Autodesk Inventor part; units mm, degrees
(part 3 of 3)
sketch "Эскиз6" plane through (0, 2, 0) normal (0, 1, 0) x (1, 0, 0)
  circle A0 centre (0, -40) radius 1.6 construction
  circle A1 centre (-46, 0) radius 1.6 construction
  circle A2 centre (46, 0) radius 1.6 construction
  line L0 (-6.2595, 46.1335) -> (-19.2746, 46.1335) construction
  arc A3 (-19.2746, 46.1335) -> (-21.6698, 47.1257) centre (-21.9203, 43.1335) ccw construction
  line L1 (-21.6698, 47.1257) -> (-42.4264, 67.8823) construction
  line L2 (-42.4264, 67.8823) -> (-34.2947, 76.014) construction
  arc A4 (-34.2947, 76.014) -> (-34.2947, 83.085) centre (-37.8302, 79.5495) ccw construction
  line L3 (-34.2947, 83.085) -> (-38.3892, 87.1795) construction
  arc A5 (-37.7453, 90.4395) -> (-38.3892, 87.1795) centre (-36.975, 88.5938) ccw construction
  arc A6 (-25.8102, 94.5401) -> (-37.7453, 90.4395) centre (0, 0) ccw construction
  arc A7 (-25.8102, 94.5401) -> (-20.7476, 95.7786) centre (-24, 98.1071) ccw construction
  arc A8 (20.7476, 95.7786) -> (-20.7476, 95.7786) centre (0, 0) ccw construction
  arc A9 (20.7476, 95.7786) -> (25.8102, 94.5401) centre (24, 98.1071) ccw construction
  arc A10 (37.7453, 90.4395) -> (25.8102, 94.5401) centre (0, 0) ccw construction
  arc A11 (38.3892, 87.1795) -> (37.7453, 90.4395) centre (36.975, 88.5938) ccw construction
  line L4 (38.3892, 87.1795) -> (34.2947, 83.085) construction
  arc A12 (34.2947, 83.085) -> (34.2947, 76.014) centre (37.8302, 79.5495) ccw construction
  line L5 (34.2947, 76.014) -> (42.4264, 67.8823) construction
  line L6 (42.4264, 67.8823) -> (21.6698, 47.1257) construction
  arc A13 (21.6698, 47.1257) -> (19.2746, 46.1335) centre (21.9203, 43.1335) ccw construction
  line L7 (19.2746, 46.1335) -> (6.2595, 46.1335) construction
  arc A14 (3.5768, 47.7906) -> (6.2595, 46.1335) centre (6.2595, 49.1335) ccw construction
  arc A15 (3.5768, 47.7906) -> (-3.5768, 47.7906) centre (0, 46) ccw construction
  arc A16 (-6.2595, 46.1335) -> (-3.5768, 47.7906) centre (-6.2595, 49.1335) ccw construction
  arc A17 (48.6481, 93.0503) -> (-48.6481, 93.0503) centre (0, 0) ccw construction
  arc A18 (-48.6481, 93.0503) -> (-49.3795, 88.2704) centre (-47.2582, 90.3917) ccw construction
  line L8 (-49.3795, 88.2704) -> (-46.3155, 85.2064) construction
  arc A19 (-46.3155, 73.8927) -> (-46.3155, 85.2064) centre (-51.9723, 79.5495) ccw construction
  line L9 (-46.3155, 73.8927) -> (-73.8927, 46.3155) construction
  arc A20 (-85.2064, 46.3155) -> (-73.8927, 46.3155) centre (-79.5495, 51.9723) ccw construction
  line L10 (-85.2064, 46.3155) -> (-88.2704, 49.3795) construction
  arc A21 (-88.2704, 49.3795) -> (-93.0503, 48.6481) centre (-90.3917, 47.2582) ccw projected
  arc A22 (-93.0503, 48.6481) -> (-93.0503, -48.6481) centre (0, 0) ccw construction
  arc A23 (-93.0503, -48.6481) -> (-88.2704, -49.3795) centre (-90.3917, -47.2582) ccw projected
  line L11 (-88.2704, -49.3795) -> (-85.2064, -46.3155) construction
  arc A24 (-73.8927, -46.3155) -> (-85.2064, -46.3155) centre (-79.5495, -51.9723) ccw construction
  line L12 (-73.8927, -46.3155) -> (-46.3155, -73.8927) construction
  arc A25 (-46.3155, -85.2064) -> (-46.3155, -73.8927) centre (-51.9723, -79.5495) ccw construction
  line L13 (-46.3155, -85.2064) -> (-49.3795, -88.2704) construction
  arc A26 (-49.3795, -88.2704) -> (-48.6481, -93.0503) centre (-47.2582, -90.3917) ccw construction
  arc A27 (-48.6481, -93.0503) -> (-45.42, -94.668) centre (0, 0) ccw construction
  arc A28 (-45.42, -94.668) -> (-43.0355, -94.1655) centre (-44.5548, -92.8648) ccw construction
  line L14 (-43.0355, -94.1655) -> (-18.3802, -65.3664) construction
  arc A29 (-17.477, -64.7643) -> (-18.3802, -65.3664) centre (-16.8609, -66.6671) ccw construction
  line L15 (-17.477, -64.7643) -> (-0.6161, -59.3045) construction
  arc A30 (0.6161, -59.3045) -> (-0.6161, -59.3045) centre (0, -61.2072) ccw construction
  line L16 (0.6161, -59.3045) -> (17.477, -64.7643) construction
  arc A31 (18.3802, -65.3664) -> (17.477, -64.7643) centre (16.8609, -66.6671) ccw construction
  line L17 (18.3802, -65.3664) -> (43.0355, -94.1655) construction
  arc A32 (43.0355, -94.1655) -> (45.42, -94.668) centre (44.5548, -92.8648) ccw construction
  arc A33 (45.42, -94.668) -> (48.6481, -93.0503) centre (0, 0) ccw construction
  arc A34 (48.6481, -93.0503) -> (49.3795, -88.2704) centre (47.2582, -90.3917) ccw construction
  line L18 (49.3795, -88.2704) -> (46.3155, -85.2064) construction
  arc A35 (46.3155, -73.8927) -> (46.3155, -85.2064) centre (51.9723, -79.5495) ccw construction
  line L19 (46.3155, -73.8927) -> (73.8927, -46.3155) construction
  arc A36 (85.2064, -46.3155) -> (73.8927, -46.3155) centre (79.5495, -51.9723) ccw construction
  line L20 (85.2064, -46.3155) -> (88.2704, -49.3795) construction
  arc A37 (88.2704, -49.3795) -> (93.0503, -48.6481) centre (90.3917, -47.2582) ccw construction
  arc A38 (93.0503, -48.6481) -> (93.0503, 48.6481) centre (0, 0) ccw construction
  arc A39 (93.0503, 48.6481) -> (88.2704, 49.3795) centre (90.3917, 47.2582) ccw construction
  line L21 (88.2704, 49.3795) -> (85.2064, 46.3155) construction
  arc A40 (73.8927, 46.3155) -> (85.2064, 46.3155) centre (79.5495, 51.9723) ccw construction
  line L22 (73.8927, 46.3155) -> (46.3155, 73.8927) construction
  arc A41 (46.3155, 85.2064) -> (46.3155, 73.8927) centre (51.9723, 79.5495) ccw construction
  line L23 (46.3155, 85.2064) -> (49.3795, 88.2704) construction
  arc A42 (49.3795, 88.2704) -> (48.6481, 93.0503) centre (47.2582, 90.3917) ccw construction
  circle A43 centre (-24, 98.1071) radius 1.6 construction
  arc A44 (47.7906, -3.5768) -> (46.1335, -6.2595) centre (49.1335, -6.2595) ccw construction
  arc A45 (47.7906, -3.5768) -> (47.7906, 3.5768) centre (46, 0) ccw construction
  arc A46 (46.1335, 6.2595) -> (47.7906, 3.5768) centre (49.1335, 6.2595) ccw construction
  line L24 (46.1335, 6.2595) -> (46.1335, 19.2746) construction
  arc A47 (46.1335, 19.2746) -> (47.1257, 21.6698) centre (43.1335, 21.9203) ccw construction
  line L25 (47.1257, 21.6698) -> (67.8823, 42.4264) construction
  line L26 (67.8823, 42.4264) -> (76.014, 34.2947) construction
  arc A48 (76.014, 34.2947) -> (83.085, 34.2947) centre (79.5495, 37.8302) ccw construction
  line L27 (83.085, 34.2947) -> (87.1795, 38.3892) construction
  arc A49 (90.4395, 37.7453) -> (87.1795, 38.3892) centre (88.5938, 36.975) ccw construction
  arc A50 (97.9653, 2.6059) -> (90.4395, 37.7453) centre (0, 0) ccw construction
  arc A51 (97.9653, 2.6059) -> (97.9653, -2.6059) centre (101, 0) ccw construction
  arc A52 (90.4395, -37.7453) -> (97.9653, -2.6059) centre (0, 0) ccw construction
  arc A53 (87.1795, -38.3892) -> (90.4395, -37.7453) centre (88.5938, -36.975) ccw construction
  line L28 (87.1795, -38.3892) -> (83.085, -34.2947) construction
  arc A54 (83.085, -34.2947) -> (76.014, -34.2947) centre (79.5495, -37.8302) ccw construction
  line L29 (76.014, -34.2947) -> (67.8823, -42.4264) construction
  line L30 (67.8823, -42.4264) -> (47.1257, -21.6698) construction
  arc A55 (47.1257, -21.6698) -> (46.1335, -19.2746) centre (43.1335, -21.9203) ccw construction
  line L31 (46.1335, -19.2746) -> (46.1335, -6.2595) construction
  circle A56 centre (101, 0) radius 1.9 construction
  circle A57 centre (-101, 0) radius 1.9 construction
  arc A58 (-47.7906, 3.5768) -> (-46.1335, 6.2595) centre (-49.1335, 6.2595) ccw construction
  arc A59 (-47.7906, 3.5768) -> (-47.7906, -3.5768) centre (-46, 0) ccw construction
  arc A60 (-46.1335, -6.2595) -> (-47.7906, -3.5768) centre (-49.1335, -6.2595) ccw construction
  line L32 (-46.1335, -6.2595) -> (-46.1335, -19.2746) construction
  arc A61 (-46.1335, -19.2746) -> (-47.1257, -21.6698) centre (-43.1335, -21.9203) ccw construction
  line L33 (-47.1257, -21.6698) -> (-67.8823, -42.4264) construction
  line L34 (-67.8823, -42.4264) -> (-76.014, -34.2947) construction
  arc A62 (-76.014, -34.2947) -> (-83.085, -34.2947) centre (-79.5495, -37.8302) ccw construction
  line L35 (-83.085, -34.2947) -> (-87.1795, -38.3892) construction
  arc A63 (-90.4395, -37.7453) -> (-87.1795, -38.3892) centre (-88.5938, -36.975) ccw construction
  arc A64 (-97.9653, -2.6059) -> (-90.4395, -37.7453) centre (0, 0) ccw construction
  arc A65 (-97.9653, -2.6059) -> (-97.9653, 2.6059) centre (-101, 0) ccw construction
  arc A66 (-90.4395, 37.7453) -> (-97.9653, 2.6059) centre (0, 0) ccw construction
  arc A67 (-87.1795, 38.3892) -> (-90.4395, 37.7453) centre (-88.5938, 36.975) ccw construction
  line L36 (-87.1795, 38.3892) -> (-83.085, 34.2947) construction
  arc A68 (-83.085, 34.2947) -> (-76.014, 34.2947) centre (-79.5495, 37.8302) ccw construction
  line L37 (-76.014, 34.2947) -> (-67.8823, 42.4264) construction
  line L38 (-67.8823, 42.4264) -> (-47.1257, 21.6698) construction
  arc A69 (-47.1257, 21.6698) -> (-46.1335, 19.2746) centre (-43.1335, 21.9203) ccw construction
  line L39 (-46.1335, 19.2746) -> (-46.1335, 6.2595) construction
  circle A70 centre (45.1111, -90.3659) radius 1.9 construction
  circle A71 centre (45.1111, 90.3659) radius 1.9 construction
  circle A72 centre (90.3659, 45.1111) radius 1.9 construction
  circle A73 centre (-45.1111, -90.3659) radius 1.9 construction
  circle A74 centre (90.3659, -45.1111) radius 1.9 construction
  circle A75 centre (-45.1111, 90.3659) radius 1.9 construction
  circle A76 centre (-90.3659, 45.1111) radius 1.9 construction
  circle A77 centre (-90.3659, -45.1111) radius 1.9 construction
  line L40 (63.6396, 46.669) -> (43.8406, 26.8701) construction
  arc A78 (41.0122, 26.8701) -> (43.8406, 26.8701) centre (42.4264, 28.2843) ccw construction
  line L41 (41.0122, 26.8701) -> (26.8701, 41.0122) construction
  arc A79 (26.8701, 43.8406) -> (26.8701, 41.0122) centre (28.2843, 42.4264) ccw construction
  line L42 (26.8701, 43.8406) -> (46.669, 63.6396) construction
  line L43 (46.669, 63.6396) -> (63.6396, 46.669) construction
  line L44 (-46.669, 63.6396) -> (-26.8701, 43.8406) construction
  arc A80 (-26.8701, 41.0122) -> (-26.8701, 43.8406) centre (-28.2843, 42.4264) ccw construction
  line L45 (-26.8701, 41.0122) -> (-41.0122, 26.8701) construction
  arc A81 (-43.8406, 26.8701) -> (-41.0122, 26.8701) centre (-42.4264, 28.2843) ccw construction
  line L46 (-43.8406, 26.8701) -> (-63.6396, 46.669) construction
  line L47 (-63.6396, 46.669) -> (-46.669, 63.6396) construction
  line L48 (-63.6396, -46.669) -> (-43.8406, -26.8701) construction
  arc A82 (-41.0122, -26.8701) -> (-43.8406, -26.8701) centre (-42.4264, -28.2843) ccw construction
  line L49 (-41.0122, -26.8701) -> (-26.8701, -41.0122) construction
  arc A83 (-26.8701, -43.8406) -> (-26.8701, -41.0122) centre (-28.2843, -42.4264) ccw construction
  line L50 (-26.8701, -43.8406) -> (-46.669, -63.6396) construction
  line L51 (-46.669, -63.6396) -> (-63.6396, -46.669) construction
  line L52 (-42.4264, -67.8823) -> (-21.6698, -47.1257) construction
  arc A84 (-21.6698, -47.1257) -> (-19.2746, -46.1335) centre (-21.9203, -43.1335) ccw construction
  line L53 (-19.2746, -46.1335) -> (19.2746, -46.1335) construction
  arc A85 (19.2746, -46.1335) -> (21.6698, -47.1257) centre (21.9203, -43.1335) ccw construction
  line L54 (21.6698, -47.1257) -> (42.4264, -67.8823) construction
  line L55 (42.4264, -67.8823) -> (37.1244, -73.1843) construction
  arc A86 (34.1909, -73.0707) -> (37.1244, -73.1843) centre (35.7102, -71.7701) ccw construction
  line L56 (34.1909, -73.0707) -> (25.4187, -62.8242) construction
  arc A87 (24.842, -61.8893) -> (25.4187, -62.8242) centre (28.1154, -60.5155) ccw construction
  line L57 (24.842, -61.8893) -> (23.8313, -59.4808) construction
  arc A88 (23.8313, -59.4808) -> (21.0049, -57.3328) centre (20.5578, -60.8546) ccw construction
  line L58 (21.0049, -57.3328) -> (15.1585, -56.5907) construction
  arc A89 (14.5119, -56.4463) -> (15.1585, -56.5907) centre (15.6055, -53.069) ccw construction
  line L59 (14.5119, -56.4463) -> (0.6161, -51.9466) construction
  arc A90 (0.6161, -51.9466) -> (-0.6161, -51.9466) centre (0, -53.8493) ccw construction
  line L60 (-0.6161, -51.9466) -> (-14.5119, -56.4463) construction
  arc A91 (-15.1585, -56.5907) -> (-14.5119, -56.4463) centre (-15.6055, -53.069) ccw construction
  line L61 (-15.1585, -56.5907) -> (-21.0049, -57.3328) construction
  arc A92 (-21.0049, -57.3328) -> (-23.8313, -59.4808) centre (-20.5578, -60.8546) ccw construction
  line L62 (-23.8313, -59.4808) -> (-24.842, -61.8893) construction
  arc A93 (-25.4187, -62.8242) -> (-24.842, -61.8893) centre (-28.1154, -60.5155) ccw construction
  line L63 (-25.4187, -62.8242) -> (-34.1909, -73.0707) construction
  arc A94 (-37.1244, -73.1843) -> (-34.1909, -73.0707) centre (-35.7102, -71.7701) ccw construction
  line L64 (-37.1244, -73.1843) -> (-42.4264, -67.8823) construction
  circle A95 centre (43.1335, 21.9203) radius 1.6 construction
  circle A96 centre (21.9203, -43.1335) radius 1.6 construction
  circle A97 centre (-21.9203, -43.1335) radius 1.6 construction
  circle A98 centre (-43.1335, -21.9203) radius 1.6 construction
  circle A99 centre (-43.1335, 21.9203) radius 1.6 construction
  circle A100 centre (-21.9203, 43.1335) radius 1.6 construction
  circle A101 centre (43.1335, -21.9203) radius 1.6 construction
  circle A102 centre (21.9203, 43.1335) radius 1.6 construction
  circle A103 centre (-37.8302, 79.5495) radius 1.6 construction
  circle A104 centre (-79.5495, 37.8302) radius 1.6 construction
  circle A105 centre (-79.5495, -37.8302) radius 1.6 construction
  circle A106 centre (79.5495, -37.8302) radius 1.6 construction
  circle A107 centre (37.8302, 79.5495) radius 1.6 construction
  circle A108 centre (79.5495, 37.8302) radius 1.6 construction
  circle A109 centre (-20.5578, -60.8546) radius 1.55 construction
  circle A110 centre (20.5578, -60.8546) radius 1.55 construction
  circle A111 centre (37.8302, -79.5495) radius 1.6 construction
  circle A112 centre (-37.8302, -79.5495) radius 1.6 construction
  line L65 (46.669, -63.6396) -> (26.8701, -43.8406) construction
  arc A113 (26.8701, -41.0122) -> (26.8701, -43.8406) centre (28.2843, -42.4264) ccw construction
  line L66 (26.8701, -41.0122) -> (41.0122, -26.8701) construction
  arc A114 (43.8406, -26.8701) -> (41.0122, -26.8701) centre (42.4264, -28.2843) ccw construction
  line L67 (43.8406, -26.8701) -> (63.6396, -46.669) construction
  line L68 (63.6396, -46.669) -> (46.669, -63.6396) construction
  circle A115 centre (24, 98.1071) radius 1.6 construction
  circle A116 centre (0, 46) radius 1.6 construction
  arc A117 (3.6492, -38.362) -> (6.3862, -40.1335) centre (6.3862, -37.1335) ccw construction
  arc A118 (3.6492, -38.362) -> (-3.6492, -38.362) centre (0, -40) ccw construction
  arc A119 (-6.3862, -40.1335) -> (-3.6492, -38.362) centre (-6.3862, -37.1335) ccw construction
  line L69 (-6.3862, -40.1335) -> (-19.2746, -40.1335) construction
  arc A120 (-19.2746, -40.1335) -> (-21.6698, -39.1414) centre (-21.9203, -43.1335) ccw construction
  line L70 (-21.6698, -39.1414) -> (-39.1414, -21.6698) construction
  arc A121 (-39.1414, -21.6698) -> (-40.1335, -19.2746) centre (-43.1335, -21.9203) ccw construction
  line L71 (-40.1335, -19.2746) -> (-40.1335, 19.2746) construction
  arc A122 (-40.1335, 19.2746) -> (-39.1414, 21.6698) centre (-43.1335, 21.9203) ccw construction
  line L72 (-39.1414, 21.6698) -> (-21.6698, 39.1414) construction
  arc A123 (-21.6698, 39.1414) -> (-19.2746, 40.1335) centre (-21.9203, 43.1335) ccw construction
  line L73 (-19.2746, 40.1335) -> (19.2746, 40.1335) construction
  arc A124 (19.2746, 40.1335) -> (21.6698, 39.1414) centre (21.9203, 43.1335) ccw construction
  line L74 (21.6698, 39.1414) -> (39.1414, 21.6698) construction
  arc A125 (39.1414, 21.6698) -> (40.1335, 19.2746) centre (43.1335, 21.9203) ccw construction
  line L75 (40.1335, 19.2746) -> (40.1335, -19.2746) construction
  arc A126 (40.1335, -19.2746) -> (39.1414, -21.6698) centre (43.1335, -21.9203) ccw construction
  line L76 (39.1414, -21.6698) -> (21.6698, -39.1414) construction
  arc A127 (21.6698, -39.1414) -> (19.2746, -40.1335) centre (21.9203, -43.1335) ccw construction
  line L77 (19.2746, -40.1335) -> (6.3862, -40.1335) construction
  arc A128 (-93.6694, -39.0933) -> (-84.7047, -40.864) centre (-88.5938, -36.975) ccw construction
  line L78 (-84.7047, -40.864) -> (-80.6102, -36.7696) construction
  arc A129 (-78.4889, -36.7696) -> (-80.6102, -36.7696) centre (-79.5495, -37.8302) ccw construction
  line L79 (-78.4889, -36.7696) -> (-67.8823, -47.3762) construction
  line L80 (-67.8823, -47.3762) -> (-42.78, -22.2739) construction
  arc A130 (-42.6335, -21.9203) -> (-42.78, -22.2739) centre (-43.1335, -21.9203) ccw construction
  line L81 (-42.6335, -21.9203) -> (-42.6335, -6.2595) construction
  line L82 (-42.6335, 6.2595) -> (-42.6335, 21.9203) construction
  arc A131 (-42.78, 22.2739) -> (-42.6335, 21.9203) centre (-43.1335, 21.9203) ccw construction
  line L83 (-42.78, 22.2739) -> (-67.8823, 47.3762) construction
  line L84 (-67.8823, 47.3762) -> (-78.4889, 36.7696) construction
  arc A132 (-80.6102, 36.7696) -> (-78.4889, 36.7696) centre (-79.5495, 37.8302) ccw construction
  line L85 (-80.6102, 36.7696) -> (-84.7047, 40.864) construction
  arc A133 (-101, -3.5) -> (-101.3693, 3.4805) centre (-101, 0) ccw
  arc A134 (-93.0503, 48.6481) -> (-93.0503, -48.6481) centre (0, 0) ccw construction
  arc A135 (-105, 0) -> (-93.0503, -48.6481) centre (0, 0) ccw
  arc A136 (-93.0503, 48.6481) -> (-105, 0) centre (0, 0) ccw
  line L86 (-88.2704, -49.3795) -> (-85.2064, -46.3155) projected
  line L87 (-90.4395, -37.7453) -> (-90.4197, -37.791)
  circle A137 centre (-101, 0) radius 1.5
  circle A138 centre (-90.3659, 45.1111) radius 1.9
  circle A139 centre (-90.3659, -45.1111) radius 1.9
  line L88 (-160.5035, 209.2939) -> (164.9125, 209.2939)
  line L89 (164.9125, 209.2939) -> (164.9125, -147.441)
  line L90 (164.9125, -147.441) -> (-160.5035, -147.441)
  line L91 (-160.5035, -147.441) -> (-160.5035, 209.2939)
  arc A140 (-89.8279, 38.5487) -> (-88.4585, -41.5951) centre (0, 0) ccw construction
  arc A141 (-93.6644, 42.8483) -> (-88.4585, 41.5951) centre (-90.3659, 45.1111) ccw
  arc A142 (-88.2704, 49.3795) -> (-93.0503, 48.6481) centre (-90.3917, 47.2582) ccw projected
  line L92 (-88.2704, 49.3795) -> (-85.7735, 46.8826)
  circle A143 centre (-46, 0) radius 1.6 construction
  line L93 (-46, 0) -> (46, 0) construction
  arc A144 (-88.4585, -41.5951) -> (-93.6644, -42.8483) centre (-90.3659, -45.1111) ccw
  arc A145 (-88.4585, 41.5951) -> (-89.8279, 38.5487) centre (0, 0) ccw construction
  arc A146 (-85.7735, 46.8826) -> (-88.4585, 41.5951) centre (0, 0) ccw
  arc A147 (-88.4585, -41.5951) -> (-85.7735, -46.8826) centre (0, 0) ccw
  arc A148 (-85.7735, -46.8826) -> (-85.7735, 46.8826) centre (0, 0) ccw construction
  arc A149 (-102.9405, -3.5) -> (-93.6644, -42.8483) centre (0, 0) ccw
  line L94 (-101, -3.5) -> (-102.9405, -3.5)
  line L95 (-46, 0) -> (-101, 0) construction
  line L96 (-101, 3.5) -> (-102.9405, 3.5)
  arc A150 (-102.9405, 3.5) -> (-102.9405, -3.5) centre (0, 0) ccw construction
  arc A151 (-93.6644, 42.8483) -> (-102.9405, 3.5) centre (0, 0) ccw
  arc A152 (-93.6644, -42.8483) -> (-93.6644, 42.8483) centre (0, 0) ccw construction
  point P0 (-101, 3.5)
  dimension "d112" = 7
  dimension "d115" = 105
  dimension "d116" = 105
  dimension "d119" = 3
  dimension "d120" = 3.8
  dimension "d121" = 3.8
  dimension "d126" = 195.5
  dimension "d128" = 4
  dimension "d139" = 2
  constraints: 44 point on circle, 36 end point, 22 centre point, 6 coincident, 4 symmetric about line, 3 horizontal, 3 parallel, 2 point on line, 1 perpendicular, 1 tangent, 12 other
  measures "d112" diameter of A133
  measures "d115" radius of A135
  measures "d116" radius of A136
  measures "d119" diameter of A137
  measures "d120" diameter of A138
  measures "d121" diameter of A139
  measures "d126" diameter of A140
  measures "d128" radius of A141
  measures "d139" radial gap between concentric circles of A22 A149
extrude "Выдавливание9" add sketch "Эскиз6" along normal blind 35 contours L92 A146 A141 A151 L96 A133 L94 A149 A144 A147 L86 A23 A135 A136 A21
extrude "Выдавливание10" cut sketch "Эскиз6" against normal blind 10 contours L92 A146 A141 A151 L96 A133 L94 A149 A144 A147 L86 A23 A135 A136 A21 | A137 | A138 | A139 | L88 L89 L90 L91
fillet "Сопряжение1" radius 2 4 edges at (-85.7735, 19.5, -46.8826) (-85.7735, 19.5, 46.8826) (-88.4585, 19.5, 41.5951) (-88.4585, 19.5, -41.5951)
ref_plane "РабПлоскость2" through (-105, 2, 0) normal (1, 0, 0) x (0, 1, 0)
sketch "Эскиз8" plane through (-105, 2, 0) normal (1, 0, 0) x (0, 1, 0)
  line L0 (0, -48.6481) -> (0, 48.6481) construction
  line L1 (0, 48.6481) -> (35, 48.6481) construction
  line L2 (35, -48.6481) -> (35, 48.6481) construction
  line L3 (0, -48.6481) -> (35, -48.6481) construction
  line L4 (0, 48.6481) -> (0, 49.3795) construction
  line L5 (0, 49.3795) -> (35, 49.3795) construction
  line L6 (35, 48.6481) -> (35, 49.3795) construction
  line L7 (0, 48.6481) -> (35, 48.6481) construction
  line L8 (0, -49.3795) -> (0, -48.6481) construction
  line L9 (0, -48.6481) -> (35, -48.6481) construction
  line L10 (35, -49.3795) -> (35, -48.6481) construction
  line L11 (0, -49.3795) -> (35, -49.3795) construction
  line L12 (0, -48.6481) -> (35, -48.6481) construction
  line L13 (0, 48.6481) -> (35, 48.6481) construction
  line L14 (35, -48.6481) -> (0, 48.6481) construction
  line L15 (35, 48.6481) -> (0, -48.6481) construction
  line L16 (11.701, 7.0442) -> (20.701, -8.5442)
  line L17 (20.701, -8.5442) -> (23.299, -7.0442)
  line L18 (23.299, -7.0442) -> (14.299, 8.5442)
  line L19 (14.299, 8.5442) -> (11.701, 7.0442)
  line L20 (11.701, 7.0442) -> (23.299, -7.0442) construction
  line L21 (20.701, -8.5442) -> (14.299, 8.5442) construction
  line L22 (35, -48.6481) -> (35, 48.6481) construction
  line L23 (35, 0) -> (0, 0) construction
  line L24 (11.701, -7.0442) -> (14.299, -8.5442)
  line L25 (23.299, 7.0442) -> (20.701, 8.5442)
  line L26 (20.701, 8.5442) -> (11.701, -7.0442)
  line L27 (14.299, -8.5442) -> (20.701, 8.5442) construction
  line L28 (23.299, 7.0442) -> (11.701, -7.0442) construction
  line L29 (14.299, -8.5442) -> (23.299, 7.0442)
  line L30 (26.5, -1.5) -> (26.5, 1.5)
  line L31 (8.5, 1.5) -> (8.5, -1.5)
  line L32 (8.5, -1.5) -> (26.5, -1.5)
  line L33 (26.5, 1.5) -> (8.5, -1.5) construction
  line L34 (8.5, 1.5) -> (26.5, -1.5) construction
  line L35 (26.5, 1.5) -> (8.5, 1.5)
  point P0 (-2, 0)
  point P1 (17.5, 0)
  point P2 (17.5, 0)
  point P3 (17.5, 0)
  point P4 (14.9019, 1.5)
  point P5 (14.9019, -1.5)
  point P6 (17.5, -3)
  point P7 (20.0981, -1.5)
  point P8 (20.0981, 1.5)
  point P9 (17.5, 3)
  dimension "d143" = 3
  dimension "d144" = 18
  dimension "d145" = 60
  dimension "d148" = 360
  constraints: 42 end point, 9 midpoint, 2 coincident, 2 parallel, 1 perpendicular, 32 other
  measures "d143" distance of L17.end L16.end
  measures "d144" distance of L17.end L18.end
  measures "d145" angle of L23 L18
extrude "Выдавливание11" cut sketch "Эскиз8" along normal blind 0.6
fillet "Сопряжение2" [suppressed]
sketch3d "3D эскиз1"
ref_plane "РабПлоскость4" through (-95, 0, 0) normal (1, 0, 0) x (0, 1, 0)
sketch "Эскиз11" plane through (-95, 0, 0) normal (1, 0, 0) x (0, 1, 0)
  line L0 (2, -3.5) -> (2, 3.5) construction
  line L1 (2, -3.5) -> (37, -3.5) construction
  line L2 (37, 3.5) -> (37, -3.5) construction
  line L3 (2, 3.5) -> (37, 3.5) construction
  line L4 (2, 3.5) -> (2, 42.8483) construction
  line L5 (2, 3.5) -> (37, 3.5) construction
  line L6 (37, 42.8483) -> (37, 3.5) construction
  line L7 (2, 42.8483) -> (37, 42.8483) construction
  line L8 (2, -42.8483) -> (2, -3.5) construction
  line L9 (2, -42.8483) -> (37, -42.8483) construction
  line L10 (37, -3.5) -> (37, -42.8483) construction
  line L11 (2, -3.5) -> (37, -3.5) construction
  line L12 (37, -48.6481) -> (37, 48.6481) construction
  line L13 (37, 0) -> (2, 0) construction
  circle A0 centre (19.5, 0) radius 13
  circle A1 centre (19.5, 0) radius 14.5
  line L14 (16.5, 22.5041) -> (16.5, -24.9376)
  point P0 (0, 0)
  point P1 (16.5, 14.1863)
  point P2 (16.5, -14.1863)
  point P3 (16.5, -12.6491)
  point P4 (16.5, 12.6491)
  dimension "d158" = 26
  dimension "d159" = 1.5
  dimension "d160" = 3
  constraints: 4 end point, 3 midpoint, 2 centre point, 1 coincident, 1 vertical, 2 other
  measures "d158" diameter of A0
  measures "d159" radial gap between concentric circles of A0 A1
  measures "d160" distance from line of A0.centre L14
extrude "Выдавливание12" add sketch "Эскиз11" against normal blind 8 contours A0 L14 A1 picked at (5.6061, 0.5258)
extrude "Выдавливание13" add sketch "Эскиз11" along normal blind 31 contours A0 L14 A1 picked at (5.6061, 0.5258)
extrude "Выдавливание14" add sketch "Эскиз11" against normal blind 2 contours L14 A0 picked at (11.9713, 2.4758)
sketch "Эскиз12" plane through (-64, 0, 0) normal (1, 0, 0) x (0, 0, -1)
  line L0 (-12.6491, 16.5) -> (-14.1863, 16.5) projected
  arc A0 (-14.1863, 16.5) -> (14.1863, 16.5) centre (0, 19.5) ccw projected
  line L1 (14.1863, 16.5) -> (12.6491, 16.5) projected
  arc A1 (-12.6491, 16.5) -> (12.6491, 16.5) centre (0, 19.5) ccw construction
  line L2 (8.9443, 20.5) -> (18.473, 20.5)
  arc A2 (-18.473, 20.5) -> (18.473, 20.5) centre (0, 19.5) ccw
  line L3 (-18.473, 20.5) -> (-8.9443, 20.5)
  arc A3 (-8.9443, 20.5) -> (8.9443, 20.5) centre (0, 19.5) ccw
  arc A4 (-12.6491, 16.5) -> (12.6491, 16.5) centre (0, 19.5) ccw construction
  line L4 (-12.6491, 16.5) -> (-8.4853, 16.5)
  line L5 (-12.6491, 16.5) -> (12.6491, 16.5) projected
  line L6 (12.6491, 16.5) -> (14.1863, 16.5) projected
  line L7 (8.4853, 16.5) -> (12.6491, 16.5)
  point P0 (0, 0)
  dimension "d167" = 4
  constraints: 8 end point, 6 point on circle, 2 centre point, 2 point on line, 1 horizontal, 3 other
  measures "d167" radial gap between concentric circles of A1 A3
extrude "Выдавливание15" add sketch "Эскиз12" along normal blind 1.5 contours L4 A3 L5 L1 A0 L0
extrude "Выдавливание16" cut sketch "Эскиз3" along normal up to surface (35 mm away) contours A93
